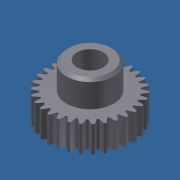
# Autodesk Inventor part: Stirnzahnrad1
Saved by Autodesk Inventor 2014 SP2 (Build 180246200, 246)
## iProperties
Created: 2014-12-14
Part Number: Stirnzahnrad1
Material: Steel
Document SubType Name: Modeling
Designer: 4ndreas
Categories: <?xml version="1.0" encoding="UTF-16"?> <MemberInstance><Categories><FamilyTemplate><FamilyTemplateParameter ValueType="xs:double" Id="1" ObjectReferenceKey="da_z" ObjectType="kUserParameterObject"/><FamilyTemplateParameter ValueType="xs:double" Id="2" ObjectReferenceKey="da_b" ObjectType="kUserParameterObject"/><FamilyTemplateParameter ValueType="xs:double" Id="3" ObjectReferenceKey="da_beta" ObjectType="kUserParameterObject"/><FamilyTemplateParameter ValueType="xs:double" Id="4" ObjectReferenceKey="da_da" ObjectType="kUserParameterObject"/><FamilyTemplateParameter ValueType="xs:double" Id="5" ObjectReferenceKey="da_aw" ObjectType="kUserParameterObject"/><FamilyTemplateParameter ValueType="xs:string" Id="6" ObjectReferenceKey="EAIAABAAAACIAQAAAAAAAIAAAAAAAAAA" ObjectType="83910656" SubObjectId="SurfaceGeometry"/></FamilyTemplate><ParamToTemplateMap><ParamToTemplate CategoryParameter="//CategoryParameter[@InternalName='046C89C9-8512-4d59-83FE-43B91F4F132A']" TemplateParameter="1"/><ParamToTemplate CategoryParameter="//CategoryParameter[@InternalName='2552DF32-E462-4b46-AEBF-C6C7768E72AC']" TemplateParameter="2"/><ParamToTemplate CategoryParameter="//CategoryParameter[@InternalName='C9EE641D-15FC-4fae-A226-E94C4372FDD7']" TemplateParameter="3"/><ParamToTemplate><ParamToTemplate CategoryParameter="//CategoryParameter[@InternalName='00B6519A-459B-49c7-AD84-2E56D39A5744']" ConstantValue="0.000000"/></ParamToTemplate><ParamToTemplate><ParamToTemplate CategoryParameter="//CategoryParameter[@InternalName='04B31F0E-C7A6-4894-AA32-9629BEFACF47']" ConstantValue="1.000000"/></ParamToTemplate><ParamToTemplate><ParamToTemplate CategoryParameter="//CategoryParameter[@InternalName='43CBEC2E-7847-49e7-A936-2F7889FCB2D9']" ConstantValue="0.250000"/></ParamToTemplate><ParamToTemplate><ParamToTemplate CategoryParameter="//CategoryParameter[@InternalName='B1EFC894-105D-4ebd-86BF-FA20ED196853']" ConstantValue="0.350000"/></ParamToTemplate><ParamToTemplate><ParamToTemplate CategoryParameter="//CategoryParameter[@InternalName='51175063-3D10-4879-93E8-6246FE8B403D']" ConstantValue="2060000000.000000"/></ParamToTemplate><ParamToTemplate><ParamToTemplate CategoryParameter="//CategoryParameter[@InternalName='A3A52E27-4454-46a9-B0BD-C932399B70AF']" ConstantValue="0.300000"/></ParamToTemplate><ParamToTemplate><ParamToTemplate CategoryParameter="//CategoryParameter[@InternalName='91B76062-C214-41d9-B1B9-14D2AB99603D']" ConstantValue="0.050000"/></ParamToTemplate><ParamToTemplate><ParamToTemplate CategoryParameter="//CategoryParameter[@InternalName='374E806E-8B8A-4dda-A9AA-1039D6500AD2']" ConstantValue="20.000000"/></ParamToTemplate><ParamToTemplate><ParamToTemplate CategoryParameter="//CategoryParameter[@InternalName='2D373A89-B862-43d6-8D0B-0CBF12AB9F6C']" ConstantValue="0.349066"/></ParamToTemplate><ParamToTemplate CategoryParameter="//CategoryParameter[@InternalName='37777632-D6A2-4fac-9D53-DB8ACD95C989']" TemplateParameter="4"/><ParamToTemplate CategoryParameter="//CategoryParameter[@InternalName='FD1017F1-B727-4f7e-9707-0F86F1FF9423']" TemplateParameter="5"/><ParamToTemplate><ParamToTemplate CategoryParameter="//CategoryParameter[@InternalName='9E1B4470-B2D3-4ff1-B813-535BB4CDF51A']" ConstantValue="3520000.000000"/></ParamToTemplate><ParamToTemplate><ParamToTemplate CategoryParameter="//CategoryParameter[@InternalName='F8452263-BFF6-458c-9FB1-07C4B99E95CD']" ConstantValue="11400000.000000"/></ParamToTemplate><ParamToTemplate><ParamToTemplate CategoryParameter="//CategoryParameter[@InternalName='3E3BB259-FD49-497f-8171-6EBC954A3479']" ConstantValue="2.000000"/></ParamToTemplate><ParamToTemplate CategoryParameter="//CategoryParameter[@InternalName='27C3BAF2-7550-4e4b-AE2C-0DB134B7D9B7']" TemplateParameter="6"/></ParamToTemplateMap><Category DisplayName="Gear" InternalName="DC85795E-93AB-48d5-8EEE-5A27447B64BD" Mnemonic="Gear"><CategoryParameter DisplayName="z" InternalName="046C89C9-8512-4d59-83FE-43B91F4F132A" Mnemonic="z"/><CategoryParameter DisplayName="b" InternalName="2552DF32-E462-4b46-AEBF-C6C7768E72AC" Mnemonic="b"/><CategoryParameter DisplayName="||b|" InternalName="C9EE641D-15FC-4fae-A226-E94C4372FDD7" Mnemonic="beta"/><CategoryParameter DisplayName="x" InternalName="00B6519A-459B-49c7-AD84-2E56D39A5744" Mnemonic="x"/><CategoryParameter DisplayName="a*" InternalName="04B31F0E-C7A6-4894-AA32-9629BEFACF47" Mnemonic="a"/><CategoryParameter DisplayName="c*" InternalName="43CBEC2E-7847-49e7-A936-2F7889FCB2D9" Mnemonic="c"/><CategoryParameter DisplayName="r|.f|*" InternalName="B1EFC894-105D-4ebd-86BF-FA20ED196853" Mnemonic="rf"/><CategoryParameter DisplayName="E" InternalName="51175063-3D10-4879-93E8-6246FE8B403D" Mnemonic="E"/><CategoryParameter DisplayName="||m|" InternalName="A3A52E27-4454-46a9-B0BD-C932399B70AF" Mnemonic="mi"/><Category DisplayName="SpurGear" InternalName="26C5A22E-A91E-4dfd-A3B3-23CCAFAE1764" Mnemonic="SpurGear"><CategoryParameter DisplayName="m" InternalName="91B76062-C214-41d9-B1B9-14D2AB99603D" Mnemonic="m"/><CategoryParameter DisplayName="P" InternalName="374E806E-8B8A-4dda-A9AA-1039D6500AD2" Mnemonic="PP"/><CategoryParameter DisplayName="||a|" InternalName="2D373A89-B862-43d6-8D0B-0CBF12AB9F6C" Mnemonic="alpha"/><CategoryParameter DisplayName="d|.a|" InternalName="37777632-D6A2-4fac-9D53-DB8ACD95C989" Mnemonic="da"/><CategoryParameter DisplayName="a|.w|" InternalName="FD1017F1-B727-4f7e-9707-0F86F1FF9423" Mnemonic="aw"/><CategoryParameter DisplayName="||s||.Flim|" InternalName="9E1B4470-B2D3-4ff1-B813-535BB4CDF51A" Mnemonic="sFlim"/><CategoryParameter DisplayName="||s||.Hlim|" InternalName="F8452263-BFF6-458c-9FB1-07C4B99E95CD" Mnemonic="sHlim"/><CategoryParameter DisplayName="Typ" InternalName="3E3BB259-FD49-497f-8171-6EBC954A3479" Mnemonic="type"/><CategoryParameter DisplayName="PitchDiameter" InternalName="27C3BAF2-7550-4e4b-AE2C-0DB134B7D9B7" Mnemonic="IDS_PITCHDIAM"/></Category></Category></Categories></MemberInstance>
Density: 7.85 g/cm^3
Appearance: Steel
Mass: 7.8085 g
Surface Area: 10.7401 cm^2
Volume: 0.994714 cm^3
CustomPartVersion: 1
Author: 4ndreas
Autodesk Inventor part; units mm, degrees
sketch "Sketch1" plane through (0, 0, 0) normal (0, 0, 1) x (1, 0, 0)
  circle A0 centre (0, 0) radius 7.9938
  dimension "d0" = 15.9876
  constraints: 1 centre point
  measures "d0" diameter of A0
extrude "Extrusion1" add sketch "Sketch1" along normal blind 5
ref_plane "Work Plane2" through (0, 0, 2.5) normal (0, 0, 1) x (1, 0, 0)
sketch "Sketch2" plane through (0, 0, 0) normal (0, 0, -1) x (-1, 0, 0)
  circle A0 centre (0, 0) radius 7.9938 projected
  circle A1 centre (0, 0) radius 7.565
  dimension "d3" = 15.1301
  constraints: 1 centre point, 1 coincident
  measures "d3" diameter of A1
surface extrude "Flankendurchmesser" sketch "Sketch2" against normal through all shown no curves A1
ref_plane "Work Plane8" through (0, 0, 0) normal (0.9945219, 0.1045285, 0) x (0, 0, 1)
ref_plane "Work Plane9" through (0, 0, 0) normal (1, 0, 0) x (0, 1, 0)
spur gear teeth "Stirnzahnrad" teeth 30 pitch diameter 15 tip diameter 15.9876 root diameter 13.75 face width 5 start plane through (0, 0, 0) normal (0, 0, -1) x (-1, 0, 0)
sketch "Skizze3" plane through (0, 0, 5) normal (0, 0, 1) x (1, 0, 0)
  circle A0 centre (0.0272, 0) radius 4.5
  arc A1 (-1.8661, 7.7729) -> (-1.9526, 6.5919) centre (3.0094, 6.8222) ccw projected
  arc A2 (-1.9526, 6.5919) -> (-2.2949, 6.4807) centre (0, 0) ccw projected
  arc A3 (-2.2949, 6.4807) -> (-3.0591, 7.3853) centre (-6.4447, 3.7504) ccw projected
  arc A4 (-3.0591, 7.3853) -> (-3.4414, 7.2151) centre (0, 0) ccw projected
  arc A5 (-3.4414, 7.2151) -> (-3.2805, 6.0419) centre (1.5252, 7.2988) ccw projected
  arc A6 (-3.2805, 6.0419) -> (-3.5922, 5.8619) centre (0, 0) ccw projected
  arc A7 (-3.5922, 5.8619) -> (-4.5277, 6.5879) centre (-7.0836, 2.3285) ccw projected
  arc A8 (-4.5277, 6.5879) -> (-4.8663, 6.3419) centre (0, 0) ccw projected
  arc A9 (-4.8663, 6.3419) -> (-4.465, 5.2278) centre (-0.0256, 7.4564) ccw projected
  arc A10 (-4.465, 5.2278) -> (-4.7324, 4.9869) centre (0, 0) ccw projected
  arc A11 (-4.7324, 4.9869) -> (-5.7985, 5.5026) centre (-7.4129, 0.8049) ccw projected
  arc A12 (-5.7985, 5.5026) -> (-6.0785, 5.1916) centre (0, 0) ccw projected
  arc A13 (-6.0785, 5.1916) -> (-5.4543, 4.1852) centre (-1.5753, 7.2882) ccw projected
  arc A14 (-5.4543, 4.1852) -> (-5.6659, 3.894) centre (0, 0) ccw projected
  arc A15 (-5.6659, 3.894) -> (-6.8158, 4.1767) centre (-7.4183, -0.754) ccw projected
  arc A16 (-6.8158, 4.1767) -> (-7.0251, 3.8143) centre (0, 0) ccw projected
  arc A17 (-7.0251, 3.8143) -> (-6.2053, 2.9598) centre (-3.0562, 6.8014) ccw projected
  arc A18 (-6.2053, 2.9598) -> (-6.3517, 2.6309) centre (0, 0) ccw projected
  arc A19 (-6.3517, 2.6309) -> (-7.5353, 2.6684) centre (-7.0994, -2.2798) ccw projected
  arc A20 (-7.5353, 2.6684) -> (-7.6646, 2.2704) centre (0, 0) ccw projected
  arc A21 (-7.6646, 2.2704) -> (-6.685, 1.6049) centre (-4.4035, 6.0173) ccw projected
  arc A22 (-6.685, 1.6049) -> (-6.7599, 1.2529) centre (0, 0) ccw projected
  arc A23 (-6.7599, 1.2529) -> (-7.9254, 1.0434) centre (-6.4703, -3.706) ccw projected
  arc A24 (-7.9254, 1.0434) -> (-7.9692, 0.6272) centre (0, 0) ccw projected
  arc A25 (-7.9692, 0.6272) -> (-6.8726, 0.18) centre (-5.5583, 4.9703) ccw projected
  arc A26 (-6.8726, 0.18) -> (-6.8726, -0.18) centre (0, 0) ccw projected
  arc A27 (-6.8726, -0.18) -> (-7.9692, -0.6272) centre (-5.5583, -4.9703) ccw projected
  arc A28 (-7.9692, -0.6272) -> (-7.9254, -1.0434) centre (0, 0) ccw projected
  arc A29 (-7.9254, -1.0434) -> (-6.7599, -1.2529) centre (-6.4703, 3.706) ccw projected
  arc A30 (-6.7599, -1.2529) -> (-6.685, -1.6049) centre (0, 0) ccw projected
  arc A31 (-6.685, -1.6049) -> (-7.6646, -2.2704) centre (-4.4035, -6.0173) ccw projected
  arc A32 (-7.6646, -2.2704) -> (-7.5353, -2.6684) centre (0, 0) ccw projected
  arc A33 (-7.5353, -2.6684) -> (-6.3517, -2.6309) centre (-7.0994, 2.2798) ccw projected
  arc A34 (-6.3517, -2.6309) -> (-6.2053, -2.9598) centre (0, 0) ccw projected
  arc A35 (-6.2053, -2.9598) -> (-7.0251, -3.8143) centre (-3.0562, -6.8014) ccw projected
  arc A36 (-7.0251, -3.8143) -> (-6.8158, -4.1767) centre (0, 0) ccw projected
  arc A37 (-6.8158, -4.1767) -> (-5.6659, -3.894) centre (-7.4183, 0.754) ccw projected
  arc A38 (-5.6659, -3.894) -> (-5.4543, -4.1852) centre (0, 0) ccw projected
  arc A39 (-5.4543, -4.1852) -> (-6.0785, -5.1916) centre (-1.5753, -7.2882) ccw projected
  arc A40 (-6.0785, -5.1916) -> (-5.7985, -5.5026) centre (0, 0) ccw projected
  arc A41 (-5.7985, -5.5026) -> (-4.7324, -4.9869) centre (-7.4129, -0.8049) ccw projected
  arc A42 (-4.7324, -4.9869) -> (-4.465, -5.2278) centre (0, 0) ccw projected
  arc A43 (-4.465, -5.2278) -> (-4.8663, -6.3419) centre (-0.0256, -7.4564) ccw projected
  arc A44 (-4.8663, -6.3419) -> (-4.5277, -6.5879) centre (0, 0) ccw projected
  arc A45 (-4.5277, -6.5879) -> (-3.5922, -5.8619) centre (-7.0836, -2.3285) ccw projected
  arc A46 (-3.5922, -5.8619) -> (-3.2805, -6.0419) centre (0, 0) ccw projected
  arc A47 (-3.2805, -6.0419) -> (-3.4414, -7.2151) centre (1.5252, -7.2988) ccw projected
  arc A48 (-3.4414, -7.2151) -> (-3.0591, -7.3853) centre (0, 0) ccw projected
  arc A49 (-3.0591, -7.3853) -> (-2.2949, -6.4807) centre (-6.4447, -3.7504) ccw projected
  arc A50 (-2.2949, -6.4807) -> (-1.9526, -6.5919) centre (0, 0) ccw projected
  arc A51 (-1.9526, -6.5919) -> (-1.8661, -7.7729) centre (3.0094, -6.8222) ccw projected
  arc A52 (-1.8661, -7.7729) -> (-1.4568, -7.8599) centre (0, 0) ccw projected
  arc A53 (-1.4568, -7.8599) -> (-0.8974, -6.8162) centre (-5.5241, -5.0083) ccw projected
  arc A54 (-0.8974, -6.8162) -> (-0.5394, -6.8538) centre (0, 0) ccw projected
  arc A55 (-0.5394, -6.8538) -> (-0.2093, -7.9911) centre (4.3621, -6.0474) ccw projected
  arc A56 (-0.2093, -7.9911) -> (0.2093, -7.9911) centre (0, 0) ccw projected
  arc A57 (0.2093, -7.9911) -> (0.5394, -6.8538) centre (-4.3621, -6.0474) ccw projected
  arc A58 (0.5394, -6.8538) -> (0.8974, -6.8162) centre (0, 0) ccw projected
  arc A59 (0.8974, -6.8162) -> (1.4568, -7.8599) centre (5.5241, -5.0083) ccw projected
  arc A60 (1.4568, -7.8599) -> (1.8661, -7.7729) centre (0, 0) ccw projected
  arc A61 (1.8661, -7.7729) -> (1.9526, -6.5919) centre (-3.0094, -6.8222) ccw projected
  arc A62 (1.9526, -6.5919) -> (2.2949, -6.4807) centre (0, 0) ccw projected
  arc A63 (2.2949, -6.4807) -> (3.0591, -7.3853) centre (6.4447, -3.7504) ccw projected
  arc A64 (3.0591, -7.3853) -> (3.4414, -7.2151) centre (0, 0) ccw projected
  arc A65 (3.4414, -7.2151) -> (3.2805, -6.0419) centre (-1.5252, -7.2988) ccw projected
  arc A66 (3.2805, -6.0419) -> (3.5922, -5.8619) centre (0, 0) ccw projected
  arc A67 (3.5922, -5.8619) -> (4.5277, -6.5879) centre (7.0836, -2.3285) ccw projected
  arc A68 (4.5277, -6.5879) -> (4.8663, -6.3419) centre (0, 0) ccw projected
  arc A69 (4.8663, -6.3419) -> (4.465, -5.2278) centre (0.0256, -7.4564) ccw projected
  arc A70 (4.465, -5.2278) -> (4.7324, -4.9869) centre (0, 0) ccw projected
  arc A71 (4.7324, -4.9869) -> (5.7985, -5.5026) centre (7.4129, -0.8049) ccw projected
  arc A72 (5.7985, -5.5026) -> (6.0785, -5.1916) centre (0, 0) ccw projected
  arc A73 (6.0785, -5.1916) -> (5.4543, -4.1852) centre (1.5753, -7.2882) ccw projected
  arc A74 (5.4543, -4.1852) -> (5.6659, -3.894) centre (0, 0) ccw projected
  arc A75 (5.6659, -3.894) -> (6.8158, -4.1767) centre (7.4183, 0.754) ccw projected
  arc A76 (6.8158, -4.1767) -> (7.0251, -3.8143) centre (0, 0) ccw projected
  arc A77 (7.0251, -3.8143) -> (6.2053, -2.9598) centre (3.0562, -6.8014) ccw projected
  arc A78 (6.2053, -2.9598) -> (6.3517, -2.6309) centre (0, 0) ccw projected
  arc A79 (6.3517, -2.6309) -> (7.5353, -2.6684) centre (7.0994, 2.2798) ccw projected
  arc A80 (7.5353, -2.6684) -> (7.6646, -2.2704) centre (0, 0) ccw projected
  arc A81 (7.6646, -2.2704) -> (6.685, -1.6049) centre (4.4035, -6.0173) ccw projected
  arc A82 (6.685, -1.6049) -> (6.7599, -1.2529) centre (0, 0) ccw projected
  arc A83 (6.7599, -1.2529) -> (7.9254, -1.0434) centre (6.4703, 3.706) ccw projected
  arc A84 (7.9254, -1.0434) -> (7.9692, -0.6272) centre (0, 0) ccw projected
  arc A85 (7.9692, -0.6272) -> (6.8726, -0.18) centre (5.5583, -4.9703) ccw projected
  arc A86 (6.8726, -0.18) -> (6.8726, 0.18) centre (0, 0) ccw projected
  arc A87 (6.8726, 0.18) -> (7.9692, 0.6272) centre (5.5583, 4.9703) ccw projected
  arc A88 (7.9692, 0.6272) -> (7.9254, 1.0434) centre (0, 0) ccw projected
  arc A89 (7.9254, 1.0434) -> (6.7599, 1.2529) centre (6.4703, -3.706) ccw projected
  arc A90 (6.7599, 1.2529) -> (6.685, 1.6049) centre (0, 0) ccw projected
  arc A91 (6.685, 1.6049) -> (7.6646, 2.2704) centre (4.4035, 6.0173) ccw projected
  arc A92 (7.6646, 2.2704) -> (7.5353, 2.6684) centre (0, 0) ccw projected
  arc A93 (7.5353, 2.6684) -> (6.3517, 2.6309) centre (7.0994, -2.2798) ccw projected
  arc A94 (6.3517, 2.6309) -> (6.2053, 2.9598) centre (0, 0) ccw projected
  arc A95 (6.2053, 2.9598) -> (7.0251, 3.8143) centre (3.0562, 6.8014) ccw projected
  arc A96 (7.0251, 3.8143) -> (6.8158, 4.1767) centre (0, 0) ccw projected
  arc A97 (6.8158, 4.1767) -> (5.6659, 3.894) centre (7.4183, -0.754) ccw projected
  arc A98 (5.6659, 3.894) -> (5.4543, 4.1852) centre (0, 0) ccw projected
  arc A99 (5.4543, 4.1852) -> (6.0785, 5.1916) centre (1.5753, 7.2882) ccw projected
  arc A100 (6.0785, 5.1916) -> (5.7985, 5.5026) centre (0, 0) ccw projected
  arc A101 (5.7985, 5.5026) -> (4.7324, 4.9869) centre (7.4129, 0.8049) ccw projected
  arc A102 (4.7324, 4.9869) -> (4.465, 5.2278) centre (0, 0) ccw projected
  arc A103 (4.465, 5.2278) -> (4.8663, 6.3419) centre (0.0256, 7.4564) ccw projected
  arc A104 (4.8663, 6.3419) -> (4.5277, 6.5879) centre (0, 0) ccw projected
  arc A105 (4.5277, 6.5879) -> (3.5922, 5.8619) centre (7.0836, 2.3285) ccw projected
  arc A106 (3.5922, 5.8619) -> (3.2805, 6.0419) centre (0, 0) ccw projected
  arc A107 (3.2805, 6.0419) -> (3.4414, 7.2151) centre (-1.5252, 7.2988) ccw projected
  arc A108 (3.4414, 7.2151) -> (3.0591, 7.3853) centre (0, 0) ccw projected
  arc A109 (3.0591, 7.3853) -> (2.2949, 6.4807) centre (6.4447, 3.7504) ccw projected
  arc A110 (2.2949, 6.4807) -> (1.9526, 6.5919) centre (0, 0) ccw projected
  arc A111 (1.9526, 6.5919) -> (1.8661, 7.7729) centre (-3.0094, 6.8222) ccw projected
  arc A112 (1.8661, 7.7729) -> (1.4568, 7.8599) centre (0, 0) ccw projected
  arc A113 (1.4568, 7.8599) -> (0.8974, 6.8162) centre (5.5241, 5.0083) ccw projected
  arc A114 (0.8974, 6.8162) -> (0.5394, 6.8538) centre (0, 0) ccw projected
  arc A115 (0.5394, 6.8538) -> (0.2093, 7.9911) centre (-4.3621, 6.0474) ccw projected
  arc A116 (0.2093, 7.9911) -> (-0.2093, 7.9911) centre (0, 0) ccw projected
  arc A117 (-0.2093, 7.9911) -> (-0.5394, 6.8538) centre (4.3621, 6.0474) ccw projected
  arc A118 (-0.5394, 6.8538) -> (-0.8974, 6.8162) centre (0, 0) ccw projected
  arc A119 (-0.8974, 6.8162) -> (-1.4568, 7.8599) centre (-5.5241, 5.0083) ccw projected
  arc A120 (-1.4568, 7.8599) -> (-1.8661, 7.7729) centre (0, 0) ccw projected
  dimension "d49" = 9
  constraints: 1 centre point
  measures "d49" diameter of A0
extrude "Extrusion2" add sketch "Skizze3" along normal blind 5 contours A0
hole "Bohrung1" at (0.0272, 0, 10) direction (0, 0, -1) diameter 5 end through all
chamfer "Fase1" distance 0.5 angle 45 1 edges at (-4.4728, 0, 10)
equation "\"d0\" = da_da"
equation "\"d1\" = da_b"
equation "\"d3\" = da_dw"
equation "\"d16\" = da_aw"
equation "\"d43\" = da_aw"
equation "\"d46\" = da_aw"
equation "\"da_da\" = 15.987596"
equation "\"da_b\" = 5"
equation "\"da_dw\" = 15.130089"
equation "\"da_aw\" = 22.695134"
body "Solid1"
body "Srf1"
